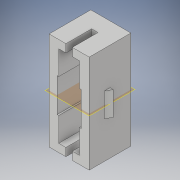
# Autodesk Inventor part: valve_body
Saved by Autodesk Inventor 2019.5 (Build 235369000, 369)
## iProperties
Created: 2021-06-12
Part Number: valve_body
Material: Generisch
Document SubType Name: Modeling
Designer: c-man
Density: 1 g/cm^3
Appearance: Vorgabe
Author: c-man
Autodesk Inventor part; units mm, degrees
ref_plane "YZ Plane" through (0, 0, 0) normal (1, 0, 0) x (0, 1, 0)
ref_plane "XZ Plane" through (0, 0, 0) normal (0, 1, 0) x (-1, 0, 0)
ref_plane "XY Plane" through (0, 0, 0) normal (0, 0, 1) x (1, 0, 0)
sketch "Skizze1" plane through (0, 0, 0) normal (0, 0, 1) x (1, 0, 0)
  line L0 (0, 0) -> (-25, 0)
  line L1 (-25, 0) -> (-25, 61)
  line L2 (-25, 61) -> (0, 61)
  line L3 (0, 61) -> (0, 0)
  dimension "d0" = 25
  dimension "d1" = 61
  constraints: 8 end point, 2 parallel, 1 horizontal, 1 perpendicular
  measures "d0" distance of L1.end L2.end
  measures "d1" distance of L0.end L1.end
extrude "Extrusion1" add sketch "Skizze1" along normal blind 26
sketch "Skizze2" plane through (0, 0, 26) normal (0, 0, 1) x (1, 0, 0)
  line L0 (-6, 56) -> (-6, 41)
  line L1 (-19, 41) -> (-19, 56)
  line L2 (0, 61) -> (-25, 61)
  line L3 (-25, 61) -> (-25, 0)
  line L4 (0, 0) -> (0, 61)
  line L5 (-6, 20) -> (-6, 5)
  line L6 (-19, 5) -> (-19, 20)
  line L7 (-25, 0) -> (0, 0)
  line L8 (-20, 41) -> (-19, 41)
  line L9 (-5, 41) -> (-5, 20)
  line L10 (-5, 20) -> (-6, 20)
  line L11 (-20, 20) -> (-20, 41)
  line L12 (-6, 41) -> (-5, 41)
  line L13 (-19, 20) -> (-20, 20)
  line L14 (-6, 5) -> (-10.5, 5)
  line L15 (-14.5, 5) -> (-19, 5)
  line L16 (-19, 56) -> (-14.5, 56)
  line L17 (-10.5, 56) -> (-6, 56)
  line L18 (-14.5, 61) -> (-10.5, 61)
  line L19 (-14.5, 0) -> (-10.5, 0)
  line L20 (-14.5, 56) -> (-10.5, 56)
  line L21 (-14.5, 5) -> (-10.5, 5)
  dimension "d4" = 25
  dimension "d5" = 13
  dimension "d6" = 6
  dimension "d7" = 13
  dimension "d8" = 5
  dimension "d9" = 5
  dimension "d10" = 21
  constraints: 44 end point, 8 parallel, 6 horizontal, 4 perpendicular, 1 point on line
  measures "d4" distance between parallel lines of L4 L3
  measures "d5" distance between parallel lines of L6 L5
  measures "d6" distance between parallel lines of L3 L6
  measures "d7" distance between parallel lines of L0 L1
  measures "d8" distance between parallel lines of L3 L11
  measures "d9" distance between parallel lines of L4 L9
  measures "d10" distance between parallel lines of L10 L8
extrude "Extrusion2" cut sketch "Skizze2" against normal blind 21 contours L0 L12 L9 L10 L5 L14 L21 L15 L6 L13 L11 L8 L1 L16 L20 L17
sketch "Skizze3" plane through (0, 0, 26) normal (0, 0, 1) x (1, 0, 0)
  line L0 (0, 61) -> (-25, 61)
  line L1 (-19, 56) -> (-6, 56)
  line L2 (-14.5, 61) -> (-10.5, 61)
  line L3 (-10.5, 61) -> (-10.5, 56)
  line L4 (-14.5, 56) -> (-14.5, 61)
  line L5 (-25, 61) -> (-25, 0)
  line L6 (0, 0) -> (0, 61)
  line L7 (-30.0841, 30.5) -> (8.1464, 30.5)
  line L8 (-14.5, 56) -> (-10.5, 56)
  line L9 (-14.5, 5) -> (-14.5, 0)
  line L10 (-10.5, 0) -> (-14.5, 0)
  line L11 (-10.5, 0) -> (-10.5, 5)
  line L12 (-14.5, 5) -> (-10.5, 5)
  point P0 (-19, 5)
  point P1 (-6, 5)
  dimension "d13" = 10.5
  dimension "d14" = 10.5
  dimension "d15" = 4
  constraints: 26 end point, 6 symmetric about line, 2 horizontal, 2 point on line, 1 collinear, 1 parallel, 1 perpendicular
  measures "d13" distance between parallel lines of L5 L4
  measures "d14" distance between parallel lines of L6 L3
  measures "d15" distance between parallel lines of L4 L3
extrude "Extrusion3" cut sketch "Skizze3" against normal blind 16 contours L3 L1 L4 L0 | L12 L11 L10 L9
ref_plane "Arbeitsebene1" through (-25, 30.5, 0) normal (0, 1, 0) x (1, 0, 0)
sketch "Skizze4" plane through (-25, 30.5, 0) normal (0, 1, 0) x (1, 0, 0)
  line L0 (14.5, -10) -> (10.5, -10) projected
  line L1 (0, 0) -> (0, -26) projected
  line L2 (0, -13) -> (-2, -13)
  line L3 (-2, -13) -> (-0.5676, -15.481)
  line L4 (-0.5676, -15.481) -> (0, -16.4641)
  line L5 (0, -13) -> (0, -16.4641)
  line L6 (25, -13) -> (27, -13)
  line L7 (27, -13) -> (25.5676, -15.481)
  line L8 (25.5676, -15.481) -> (25, -16.4641)
  line L9 (25, -13) -> (25, -16.4641)
  line L10 (0, 0) -> (25, 0) projected
  line L11 (25, -26) -> (14.5, -26) projected
  dimension "d18" = 2
  dimension "d19" = 60
  dimension "d22" = 13
  dimension "d23" = 9.5359
  dimension "d24" = 26
  constraints: 16 end point, 1 collinear, 1 horizontal, 1 midpoint, 1 point on line
  measures "d18" distance of L2.start L2.end
  measures "d19" angle of L3 L2
  measures "d22" distance between parallel lines of L6 L10
  measures "d23" distance from line of L11 L8.end
  measures "d24" distance between parallel lines of L11 L10
extrude "Extrusion4" add sketch "Skizze4" along normal mid plane 15
